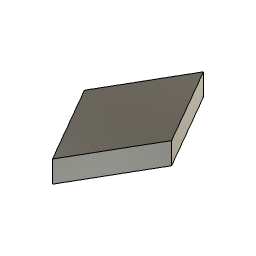
Parallelogram (Autodesk Fusion 360 design; units mm, degrees)
Autodesk Fusion 360 part; units mm, degrees
sketch "Parallelogram" plane through (0, 0, 0) normal (0, 0, 1) x (1, 0, 0)
  line L0 (6.35, 0) -> (12.7, -10.9977)
  line L1 (12.7, -10.9977) -> (6.35, -21.9964)
  line L2 (0, -10.9982) -> (6.35, 0)
  line L3 (6.35, -21.9964) -> (0, -10.9982)
extrude "Extrude1" add sketch "Parallelogram" along normal blind 3.175
